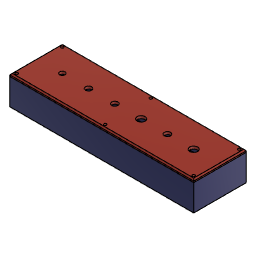
Hammond_LineOut_Headphone_Panel (Autodesk Fusion 360 design; units mm, degrees)
Autodesk Fusion 360 part; units mm, degrees
note: some values were not read from the file. Set by a fixed rule: the direction of a hole.
sketch "panel" plane through (0, 0, 0) normal (0, 0, 1) x (1, 0, 0)
  line L0 (101, -26) -> (-101, -26) construction
  line L1 (-101, -26) -> (-101, 26) construction
  line L2 (-101, 26) -> (101, 26) construction
  line L3 (101, 26) -> (101, -26) construction
  line L4 (101, -26) -> (-101, 26) construction
  line L5 (-101, -26) -> (101, 26) construction
  line L6 (105, -30) -> (-105, -30)
  line L7 (-105, -30) -> (-105, 30)
  line L8 (-105, 30) -> (105, 30)
  line L9 (105, 30) -> (105, -30)
  line L10 (105, -30) -> (-105, 30) construction
  line L11 (-105, -30) -> (105, 30) construction
  line L12 (-105, 0) -> (-75, 0) construction
  point P0 (-101, 26)
  point P1 (-101, -26)
  point P2 (101, -26)
  point P3 (101, 26)
  point P4 (0, 26)
  point P5 (0, -26)
  point P6 (-45, 0)
  point P7 (-15, 0)
  point P8 (15, 0)
  point P9 (45, 0)
  point P10 (75, 0)
  dimension "d9" = 202
  dimension "d10" = 52
  dimension "d49" = 210
  dimension "d50" = 60
  dimension "d51" = 30
  dimension "d98" = 30
  dimension "d99" = 30
  constraint horizontal L0
  constraint perpendicular L0 L1
  constraint parallel L0 L2
  constraint parallel L1 L3
  constraint coincident L4 origin
  constraint coincident L5 origin
  constraint horizontal L6
  constraint perpendicular L6 L7
  constraint parallel L6 L8
  constraint parallel L7 L9
  constraint coincident L10 origin
  constraint coincident L11 origin
  constraint coincident P0 L1.end
  constraint coincident P1 L0.end
  constraint coincident P2 L0.start
  constraint coincident P3 L2.end
  constraint midpoint L2 P4
  constraint midpoint L0 P5
  constraint midpoint L7 L12.start
  constraint perpendicular L1 L12
  measures "d9" distance of P0 L2.end
  measures "d10" distance of P1 P0
  measures "d49" distance of L7.end L8.end
  measures "d50" distance of L6.end L7.end
  measures "d51" distance of L12.start L12.end
extrude "Extrude1" add sketch "panel" along normal blind 3 makes body 1
chamfer "Chamfer1" distance 1.5 angle 45 1 faces at (-35, 10, 3) on bodies 1
hole "Hole8" at (-101, 26, 0) direction (0, 0, 1) diameter 3 end through all bodies 1
hole "Hole9" at (0, 26, 0) direction (0, 0, 1) diameter 3 end through all bodies 1
hole "Hole10" at (101, 26, 0) direction (0, 0, 1) diameter 3 end through all bodies 1
hole "Hole11" at (0, -26, 0) direction (0, 0, 1) diameter 3 end through all bodies 1
hole "Hole12" at (-101, -26, 0) direction (0, 0, 1) diameter 3 end through all bodies 1
hole "Hole13" at (101, -26, 0) direction (0, 0, 1) diameter 3 end through all bodies 1
sketch "Labels" plane through (0, 0, 0) normal (0, 0, 1) x (1, 0, 0)
  line L0 (0, 0) -> (0, -15) construction
  line L1 (0, -15) -> (0, 0) construction
  line L2 (0, -15) -> (100.1632, -15) construction
  line L3 (0, -15) -> (-91.0813, -15) construction
  line L4 (-75.1866, -16.7158) -> (-74.7316, -16.7237) construction
  line L5 (-74.7316, -16.7237) -> (-74.7043, -15.167) construction
  line L6 (-74.7043, -15.167) -> (-75.1594, -15.1591) construction
  line L7 (-75.1594, -15.1591) -> (-75.1866, -16.7158) construction
  line L8 (-45.0021, -20.9561) -> (-44.8617, -20.9538) construction
  line L9 (-44.8617, -20.9538) -> (-44.9531, -15.4379) construction
  line L10 (-44.9531, -15.4379) -> (-45.0935, -15.4402) construction
  line L11 (-45.0935, -15.4402) -> (-45.0021, -20.9561) construction
  line L12 (-14.9298, -20.9952) -> (-14.9293, -20.9952) construction
  line L13 (-14.9293, -20.9952) -> (-14.9293, -15.7293) construction
  line L14 (-14.9293, -15.7293) -> (-14.9298, -15.7293) construction
  line L15 (-14.9298, -15.7293) -> (-14.9298, -20.9952) construction
  line L16 (15.0882, -20.9952) -> (15.1001, -20.9952) construction
  line L17 (15.1001, -20.9952) -> (15.1001, -15.7293) construction
  line L18 (15.1001, -15.7293) -> (15.0882, -15.7293) construction
  line L19 (15.0882, -15.7293) -> (15.0882, -20.9952) construction
  line L20 (45.5193, -20.4126) -> (45.5312, -20.4126) construction
  line L21 (45.5312, -20.4126) -> (45.5312, -15.1467) construction
  line L22 (45.5312, -15.1467) -> (45.5193, -15.1467) construction
  line L23 (45.5193, -15.1467) -> (45.5193, -20.4126) construction
  line L24 (75.0517, -20.6068) -> (75.0636, -20.6068) construction
  line L25 (75.0636, -20.6068) -> (75.0636, -15.3409) construction
  line L26 (75.0636, -15.3409) -> (75.0517, -15.3409) construction
  line L27 (75.0517, -15.3409) -> (75.0517, -20.6068) construction
  point P0 (-20.7806, -22.7685)
  dimension "d70" = 15
  dimension "d72" = 1.5
  dimension "d76" = 1.5
  dimension "d78" = 1.5
  dimension "d79" = 1.5
  dimension "d80" = 1.5
  dimension "d81" = 1.5
  constraint coincident L0.start L1.end
  constraint vertical L0
  constraint parallel L0 L1
  constraint perpendicular L1 L2
  constraint perpendicular L0 L3
  measures "d70" distance of L0.end L0.start
hole "Hole16" at (-75, 0, 0) direction (0, 0, 1) diameter 6 end through all bodies 1
hole "Hole17" at (-45, 0, 0) direction (0, 0, 1) diameter 7 end through all bodies 1
hole "Hole18" at (-15, 0, 0) direction (0, 0, 1) diameter 7 end through all bodies 1
hole "Hole19" at (15, 0, 0) direction (0, 0, 1) diameter 9 end through all bodies 1
hole "Hole20" at (45, 0, 0) direction (0, 0, 1) diameter 7 end through all bodies 1
hole "Hole21" at (75, 0, 0) direction (0, 0, 1) diameter 9 end through all bodies 1
sketch "box" plane through (0, 0, 0) normal (0, 0, 1) x (1, 0, 0)
  line L0 (105, 30) -> (-105, 30)
  line L1 (-105, 30) -> (-105, -30)
  line L2 (-105, -30) -> (105, -30)
  line L3 (105, -30) -> (105, 30)
  line L4 (105, 30) -> (-105, -30) construction
  line L5 (-105, 30) -> (105, -30) construction
  dimension "d119" = 210
  dimension "d120" = 60
  constraint horizontal L0
  constraint perpendicular L0 L1
  constraint parallel L0 L2
  constraint parallel L1 L3
  constraint coincident L4 origin
  constraint coincident L5 origin
  measures "d119" distance of L1.end L2.end
  measures "d120" distance of L0.end L1.end
extrude "Extrude2" add sketch "box" along normal blind 30 thin wall 3 inside separate body makes body 2
cylinder "CylinderPrimitive1" add diameter 6 height 30 placed x (1, 0, 0) y (0, 1, 0) z (0, 0, 1) at (-100.9216, 26.0443, 0) bodies 2
cylinder "CylinderPrimitive2" add diameter 6 height 30 placed x (1, 0, 0) y (0, 1, 0) z (0, 0, 1) at (-101.0374, -25.9989, 0) bodies 2
cylinder "CylinderPrimitive3" add diameter 6 height 30 placed x (1, 0, 0) y (0, 1, 0) z (0, 0, 1) at (100.9153, 25.922, 0) bodies 2
cylinder "CylinderPrimitive4" add diameter 6 height 30 placed x (1, 0, 0) y (0, 1, 0) z (0, 0, 1) at (101.0304, -25.9582, 0) bodies 2
cylinder "CylinderPrimitive5" add diameter 6 height 30 placed x (1, 0, 0) y (0, 1, 0) z (0, 0, 1) at (0.1155, 25.9959, 0) bodies 2
cylinder "CylinderPrimitive6" add diameter 6 height 30 placed x (1, 0, 0) y (0, 1, 0) z (0, 0, 1) at (0.1272, -26.0192, 0) bodies 2
hole "Hole22" at (101, 26, 0) at (0, 26, 0) at (-101, 26, 0) at (-101, -26, 0) at (0, -26, 0) at (101, -26, 0) direction (0, 0, 1) diameter 1.5 depth 30 tip angle 180 bodies 2
copy_body "Body->Comp1" bodies 1 removing the originals makes body 3 in component "panel"
copy_body "Body->Comp2" bodies 2 removing the originals makes body 4 in component "box"
extrude "Extrude1'" add sketch "box" along normal blind 3 bodies 4 in component "box"
component "panel" placed x (1, 0, 0) y (0, 1, 0) z (0, 0, 1) at (0, 0, 30)
component "box" placed x (1, 0, 0) y (0, 1, 0) z (0, 0, 1) at (0, 0, 0)
equation "distance_between_holes = 30 mm"
equation "number_of_holes = 6"
equation "hole_to_edge = distance_between_holes"
equation "d9 = ( ( number_of_holes - 1 ) * distance_between_holes ) + ( 2 * hole_to_edge ) - ( 2 * mounting_hole_from_edge )"
equation "d10 = ( 2 * hole_to_edge ) - ( 2 * mounting_hole_from_edge )"
equation "pot_hole = 7 mm"
equation "small_headphone_jack_hole = 6 mm"
equation "quarter_inch_jack_hole = 9 mm"
equation "panel_thickness = 3 mm"
equation "d20 = panel_thickness"
equation "d22 = panel_thickness / 2"
equation "switch_hole = 6 mm"
equation "mounting_hole_from_edge = 4 mm"
equation "mounting_hole = 3 mm"
equation "d49 = ( ( number_of_holes - 1 ) * distance_between_holes ) + ( 2 * hole_to_edge )"
equation "d50 = ( 2 * hole_to_edge )"
equation "d51 = hole_to_edge"
equation "d53 = mounting_hole"
equation "d56 = mounting_hole"
equation "d59 = mounting_hole"
equation "d62 = mounting_hole"
equation "d65 = mounting_hole"
equation "d68 = mounting_hole"
equation "d70 = hole_to_edge / 2"
equation "d96 = number_of_holes"
equation "d98 = distance_between_holes"
equation "d99 = distance_between_holes"
equation "d101 = switch_hole"
equation "d104 = pot_hole"
equation "d110 = quarter_inch_jack_hole"
equation "d113 = pot_hole"
equation "d116 = quarter_inch_jack_hole"
equation "box_height = 30 mm"
equation "d119 = ( ( number_of_holes - 1 ) * distance_between_holes ) + ( 2 * hole_to_edge )"
equation "d120 = ( 2 * hole_to_edge )"
equation "d121 = panel_thickness"
equation "d122 = box_height"
equation "d124 = box_height"
equation "d125 = mounting_hole * 2"
equation "d126 = box_height"
equation "d128 = box_height"
equation "d129 = mounting_hole * 2"
equation "d130 = box_height"
equation "d131 = mounting_hole * 2"
equation "d132 = box_height"
equation "d133 = mounting_hole * 2"
equation "d134 = box_height"
equation "d135 = mounting_hole * 2"
equation "d136 = box_height"
equation "d137 = mounting_hole / 2"
equation "d144 = box_height"
equation "d146 = panel_thickness"
named bodies: "panel", "box"
